Autodesk Inventor part; units mm, degrees
(part 2 of 2)
  arc A292 (23.8053, 31.1147) -> (23.1322, 30.5755) centre (29.291, 23.5772) ccw projected
  arc A293 (23.1322, 30.5755) -> (21.9307, 31.4483) centre (0, 0) ccw projected
  arc A294 (21.9307, 31.4483) -> (22.2356, 32.2552) centre (13.3718, 35.1431) ccw projected
  arc A295 (22.2356, 32.2552) -> (22.5669, 33.4681) centre (9.9788, 36.2544) ccw projected
  arc A296 (22.5669, 33.4681) -> (22.8546, 35.1883) centre (6.2739, 37.0778) ccw projected
  arc A297 (22.8546, 35.1883) -> (20.9772, 36.3388) centre (0, 0) ccw projected
  arc A298 (20.9772, 36.3388) -> (19.5752, 35.3014) centre (30.1882, 22.4231) ccw projected
  arc A299 (19.5752, 35.3014) -> (18.6448, 34.4556) centre (27.7726, 25.3503) ccw projected
  arc A300 (18.6448, 34.4556) -> (18.0643, 33.8177) centre (25.2421, 27.869) ccw projected
  arc A301 (18.0643, 33.8177) -> (16.7411, 34.4919) centre (0, 0) ccw projected
  arc A302 (16.7411, 34.4919) -> (16.916, 35.3365) centre (7.7096, 36.8023) ccw projected
  arc A303 (16.916, 35.3365) -> (17.0535, 36.5863) centre (4.1845, 37.3691) ccw projected
  arc A304 (17.0535, 36.5863) -> (17.0686, 38.3303) centre (0.3965, 37.6027) ccw projected
  arc A305 (17.0686, 38.3303) -> (15.0343, 39.1729) centre (0, 0) ccw projected
  arc A306 (15.0343, 39.1729) -> (13.8118, 37.9291) centre (26.3088, 26.8695) ccw projected
  arc A307 (13.8118, 37.9291) -> (13.0252, 36.9481) centre (23.4651, 29.3828) ccw projected
  arc A308 (13.0252, 36.9481) -> (12.5517, 36.2272) centre (20.5717, 31.4746) ccw projected
  arc A309 (12.5517, 36.2272) -> (11.1393, 36.6861) centre (0, 0) ccw projected
  arc A310 (11.1393, 36.6861) -> (11.1799, 37.5477) centre (1.8575, 37.5552) ccw projected
  arc A311 (11.1799, 37.5477) -> (11.1201, 38.8036) centre (-1.7129, 37.5636) ccw projected
  arc A312 (11.1201, 38.8036) -> (10.8623, 40.5285) centre (-5.4908, 37.2018) ccw projected
  arc A313 (10.8623, 40.5285) -> (8.7212, 41.0425) centre (0, 0) ccw projected
  arc A314 (8.7212, 41.0425) -> (7.7084, 39.6227) centre (21.7816, 30.6543) ccw projected
  arc A315 (7.7084, 39.6227) -> (7.0849, 38.5308) centre (18.5797, 32.6918) ccw projected
  arc A316 (7.0849, 38.5308) -> (6.73, 37.7447) centre (15.3947, 34.3052) ccw projected
  arc A317 (6.73, 37.7447) -> (5.2632, 37.977) centre (0, 0) ccw projected
  arc A318 (5.2632, 37.977) -> (5.1685, 38.8343) centre (-4.0403, 37.3834) ccw projected
  arc A319 (5.1685, 38.8343) -> (4.9158, 40.0547) centre (-7.568, 36.8332) ccw projected
  arc A320 (4.9158, 40.0547) -> (4.3885, 41.7288) centre (-11.2428, 35.8848) ccw projected
  arc A321 (4.3885, 41.7288) -> (2.1934, 41.9015) centre (0, 0) ccw projected
  arc A322 (2.1934, 41.9015) -> (1.4107, 40.3306) centre (16.718, 33.6843) ccw projected
  arc A323 (1.4107, 40.3306) -> (0.9701, 39.1647) centre (13.2368, 35.1958) ccw projected
  arc A324 (0.9701, 39.1647) -> (0.7425, 38.3328) centre (9.8386, 36.2911) ccw projected
  circle A325 centre (50, 0) radius 9
  line L1 (0, 0) -> (50, 0) construction
  circle A326 centre (50, 4.5) radius 2
  circle A327 centre (50, -4.5) radius 2
  line L2 (50, 4.5) -> (50, -4.5)
  line L3 (0, 0) -> (34.0976, 51.9877)
  line L4 (0, 0) -> (-5.7443, -48.4608)
  line L5 (21.9307, 31.4483) -> (2.9609, 2.5256)
  line L6 (-0.7425, -38.3328) -> (3.5093, -2.4629)
  line L7 (-0.7425, -38.3328) -> (7.758, -21.4754)
  line L8 (21.9307, 31.4483) -> (18.4149, 16.5287)
  line L9 (18.4149, 16.5287) -> (52.0246, 8.7693)
  line L10 (7.758, -21.4754) -> (52.4807, -8.6514)
  point P0 (37.977, 5.2632)
  point P1 (37.0268, -13.0827)
  point P2 (36.2778, 12.4048)
  point P3 (37.7447, 6.73)
  dimension "d2" = 6
  dimension "d3" = 6.13
  dimension "d5" = 7
  dimension "d37" = 18
  dimension "d38" = 50
  dimension "d39" = 4
  dimension "d40" = 4
  dimension "d42" = 9
  dimension "d43" = 56.74
  dimension "d44" = 153.5
  dimension "d45" = 20
  dimension "d46" = 20
  dimension "d47" = 13
  dimension "d48" = 16
  constraints: 22 end point, 6 centre point, 3 point on circle, 2 coincident, 2 parallel, 2 tangent, 2 vertical, 1 horizontal, 1 midpoint, 1 vertical alignment
  measures "d2" diameter of A0
  measures "d3" radial gap between concentric circles of A1 A2
  measures "d5" radial gap between concentric circles of A0 A3
  measures "d37" diameter of A325
  measures "d38" distance of L1.end L1.start
  measures "d39" diameter of A326
  measures "d40" diameter of A327
  measures "d42" distance of L2.start L2.end
  measures "d43" angle of L1 L3
  measures "d44" angle of L4 L3
  measures "d45" angle of L6 L7
  measures "d46" angle of L5 L8
  measures "d47" angle of L1 L9
  measures "d48" angle of L10 L1
extrude "押し出し6" cut sketch "Sketch2" against normal through all contours A0 L4 L3 | L3 L4 A0 | L8 A293 A292 A291 A290 A289 A288 A287 A286 A285 A284 A283 A282 A281 A280 A279 A278 A277 A276 A275 A274 A273 A272 A271 A270 A269 A268 A267 A266 A265 A264 A263 A262 A261 L9 A1 | A1 L9 L8 | L7 L10 A1 | A1 L10 A227 A226 A225 A224 A223 A222 A221 A220 A219 A218 A217 A216 A215 A214 A213 A212 A211 A210 A209 A208 A207 A206 A205 A204 A203 A202 A201 A200 A199 A198 A197 A196 A195 A194 A193 A192 A191 A190 A189 A188 A187 A186 A185 A184 A183 A182 A181 A180 A179 A178 A177 A176 A175 A174 A173 A172 A171 A170 A169 A168 A167 A166 A165 L7
extrude "押し出し7" add sketch "Sketch2" against normal blind 4 contours L9 A325 A249 A250 A251 A252 A4 A254 A255 A256 A257 A258 A259 A260 A261 | A227 A228 A229 A230 A231 A232 A233 A234 A235 A236 A237 A238 A239 A240 A241 A325 L10 | A325 A241 A242 A248 A249 | A325 A242 A243 A244 A245 A246 A247 A248
sketch "スケッチ6" plane through (0, 0, -4) normal (0, 0, -1) x (-1, 0, 0)
  circle A0 centre (-50, 4.5) radius 2 projected
  circle A1 centre (-50, -4.5) radius 2 projected
  line L0 (-7.758, -21.4754) -> (0.7425, -38.3328) projected
  arc A2 (0.7425, -38.3328) -> (0.9701, -39.1647) centre (9.8386, -36.2911) ccw projected
  arc A3 (0.9701, -39.1647) -> (1.4151, -40.3408) centre (13.2368, -35.1958) ccw projected
  arc A4 (1.4151, -40.3408) -> (2.1934, -41.9015) centre (16.718, -33.6843) ccw projected
  arc A5 (2.1934, -41.9015) -> (4.3885, -41.7288) centre (0, 0) ccw projected
  arc A6 (4.3885, -41.7288) -> (4.913, -40.0655) centre (-11.2428, -35.8848) ccw projected
  arc A7 (4.913, -40.0655) -> (5.1685, -38.8343) centre (-7.568, -36.8332) ccw projected
  arc A8 (5.1685, -38.8343) -> (5.2632, -37.977) centre (-4.0403, -37.3834) ccw projected
  arc A9 (5.2632, -37.977) -> (6.73, -37.7447) centre (0, 0) ccw projected
  arc A10 (6.73, -37.7447) -> (7.0849, -38.5308) centre (15.3947, -34.3052) ccw projected
  arc A11 (7.0849, -38.5308) -> (7.7084, -39.6227) centre (18.5797, -32.6918) ccw projected
  arc A12 (7.7084, -39.6227) -> (8.7212, -41.0425) centre (21.7816, -30.6543) ccw projected
  arc A13 (8.7212, -41.0425) -> (10.8623, -40.5285) centre (0, 0) ccw projected
  arc A14 (10.8623, -40.5285) -> (11.1201, -38.8036) centre (-5.4908, -37.2018) ccw projected
  arc A15 (11.1201, -38.8036) -> (11.1799, -37.5477) centre (-1.7129, -37.5636) ccw projected
  arc A16 (11.1799, -37.5477) -> (11.1393, -36.6861) centre (1.8575, -37.5552) ccw projected
  arc A17 (11.1393, -36.6861) -> (12.5517, -36.2272) centre (0, 0) ccw projected
  arc A18 (12.5517, -36.2272) -> (13.0252, -36.9481) centre (20.5717, -31.4746) ccw projected
  arc A19 (13.0252, -36.9481) -> (13.8118, -37.9291) centre (23.4651, -29.3828) ccw projected
  arc A20 (13.8118, -37.9291) -> (15.0343, -39.1729) centre (26.3088, -26.8695) ccw projected
  arc A21 (15.0343, -39.1729) -> (17.0686, -38.3303) centre (0, 0) ccw projected
  arc A22 (17.0686, -38.3303) -> (17.0535, -36.5863) centre (0.3965, -37.6027) ccw projected
  arc A23 (17.0535, -36.5863) -> (16.916, -35.3365) centre (4.1845, -37.3691) ccw projected
  arc A24 (16.916, -35.3365) -> (16.7411, -34.4919) centre (7.7096, -36.8023) ccw projected
  arc A25 (16.7411, -34.4919) -> (18.0643, -33.8177) centre (0, 0) ccw projected
  arc A26 (18.0643, -33.8177) -> (18.6448, -34.4556) centre (25.2421, -27.869) ccw projected
  arc A27 (18.6448, -34.4556) -> (19.5752, -35.3014) centre (27.7726, -25.3503) ccw projected
  arc A28 (19.5752, -35.3014) -> (20.9772, -36.3388) centre (30.1882, -22.4231) ccw projected
  arc A29 (20.9772, -36.3388) -> (22.8546, -35.1883) centre (0, 0) ccw projected
  arc A30 (22.8546, -35.1883) -> (22.5669, -33.4681) centre (6.2739, -37.0778) ccw projected
  arc A31 (22.5669, -33.4681) -> (22.2356, -32.2552) centre (9.9788, -36.2544) ccw projected
  arc A32 (22.2356, -32.2552) -> (21.9307, -31.4483) centre (13.3718, -35.1431) ccw projected
  arc A33 (21.9307, -31.4483) -> (23.1322, -30.5754) centre (0, 0) ccw projected
  arc A34 (23.1322, -30.5754) -> (23.8053, -31.1147) centre (29.291, -23.5771) ccw projected
  arc A35 (23.8053, -31.1147) -> (24.8565, -31.8046) centre (31.3964, -20.6936) ccw projected
  arc A36 (24.8565, -31.8046) -> (26.4036, -32.6098) centre (33.3243, -17.4245) ccw projected
  arc A37 (26.4036, -32.6098) -> (28.0779, -31.1798) centre (0, 0) ccw projected
  arc A38 (28.0779, -31.1798) -> (27.5246, -29.5259) centre (11.9969, -35.6398) ccw projected
  arc A39 (27.5246, -29.5259) -> (27.0076, -28.3796) centre (15.5273, -34.247) ccw projected
  arc A40 (27.0076, -28.3796) -> (26.5803, -27.6304) centre (18.7048, -32.6187) ccw projected
  arc A41 (26.5803, -27.6304) -> (27.6304, -26.5803) centre (0, 0) ccw projected
  arc A42 (27.6304, -26.5803) -> (28.3796, -27.0076) centre (32.6187, -18.7048) ccw projected
  arc A43 (28.3796, -27.0076) -> (29.5259, -27.5246) centre (34.247, -15.5273) ccw projected
  arc A44 (29.5259, -27.5246) -> (31.1798, -28.0779) centre (35.6398, -11.9969) ccw projected
  arc A45 (31.1798, -28.0779) -> (32.6098, -26.4036) centre (0, 0) ccw projected
  arc A46 (32.6098, -26.4036) -> (31.8046, -24.8565) centre (17.4245, -33.3243) ccw projected
  arc A47 (31.8046, -24.8565) -> (31.1147, -23.8053) centre (20.6936, -31.3964) ccw projected
  arc A48 (31.1147, -23.8053) -> (30.5754, -23.1322) centre (23.5771, -29.291) ccw projected
  arc A49 (30.5754, -23.1322) -> (31.4483, -21.9307) centre (0, 0) ccw projected
  arc A50 (31.4483, -21.9307) -> (32.2552, -22.2356) centre (35.1431, -13.3718) ccw projected
  arc A51 (32.2552, -22.2356) -> (33.4681, -22.5669) centre (36.2544, -9.9788) ccw projected
  arc A52 (33.4681, -22.5669) -> (35.1883, -22.8546) centre (37.0778, -6.2739) ccw projected
  arc A53 (35.1883, -22.8546) -> (36.3388, -20.9772) centre (0, 0) ccw projected
  arc A54 (36.3388, -20.9772) -> (35.3014, -19.5752) centre (22.4231, -30.1882) ccw projected
  arc A55 (35.3014, -19.5752) -> (34.4556, -18.6448) centre (25.3503, -27.7726) ccw projected
  arc A56 (34.4556, -18.6448) -> (33.8177, -18.0643) centre (27.869, -25.2421) ccw projected
  arc A57 (33.8177, -18.0643) -> (34.4919, -16.7411) centre (0, 0) ccw projected
  arc A58 (34.4919, -16.7411) -> (35.3365, -16.916) centre (36.8023, -7.7096) ccw projected
  arc A59 (35.3365, -16.916) -> (36.5863, -17.0535) centre (37.3691, -4.1845) ccw projected
  arc A60 (36.5863, -17.0535) -> (38.3303, -17.0686) centre (37.6027, -0.3965) ccw projected
  arc A61 (38.3303, -17.0686) -> (39.1729, -15.0343) centre (0, 0) ccw projected
  arc A62 (39.1729, -15.0343) -> (37.9291, -13.8118) centre (26.8695, -26.3088) ccw projected
  arc A63 (37.9291, -13.8118) -> (36.9481, -13.0252) centre (29.3828, -23.4651) ccw projected
  arc A64 (36.9481, -13.0252) -> (36.2272, -12.5517) centre (31.4746, -20.5717) ccw projected
  arc A65 (36.2272, -12.5517) -> (36.6861, -11.1393) centre (0, 0) ccw projected
  arc A66 (36.6861, -11.1393) -> (37.5477, -11.1799) centre (37.5552, -1.8575) ccw projected
  arc A67 (37.5477, -11.1799) -> (38.7926, -11.1212) centre (37.5636, 1.7129) ccw projected
  arc A68 (38.7926, -11.1212) -> (40.5285, -10.8623) centre (37.2018, 5.4908) ccw projected
  arc A69 (40.5285, -10.8623) -> (41.0425, -8.7212) centre (0, 0) ccw projected
  arc A70 (41.0425, -8.7212) -> (39.6227, -7.7084) centre (30.6543, -21.7816) ccw projected
  arc A71 (39.6227, -7.7084) -> (38.5308, -7.0849) centre (32.6918, -18.5797) ccw projected
  arc A72 (38.5308, -7.0849) -> (37.7447, -6.73) centre (34.3052, -15.3947) ccw projected
  arc A73 (37.7447, -6.73) -> (37.977, -5.2632) centre (0, 0) ccw projected
  arc A74 (37.977, -5.2632) -> (38.8343, -5.1685) centre (37.3834, 4.0403) ccw projected
  arc A75 (38.8343, -5.1685) -> (40.0655, -4.913) centre (36.8332, 7.568) ccw projected
  arc A76 (40.0655, -4.913) -> (41.7288, -4.3885) centre (35.8848, 11.2428) ccw projected
  arc A77 (41.7288, -4.3885) -> (41.9015, -2.1934) centre (0, 0) ccw projected
  arc A78 (41.9015, -2.1934) -> (40.3306, -1.4107) centre (33.6843, -16.718) ccw projected
  arc A79 (40.3306, -1.4107) -> (39.1647, -0.9701) centre (35.1958, -13.2368) ccw projected
  arc A80 (39.1647, -0.9701) -> (38.3328, -0.7425) centre (36.2911, -9.8386) ccw projected
  arc A81 (38.3328, -0.7425) -> (38.3328, 0.7425) centre (0, 0) ccw projected
  arc A82 (38.3328, 0.7425) -> (39.1647, 0.9701) centre (36.2911, 9.8386) ccw projected
  arc A83 (39.1647, 0.9701) -> (40.3306, 1.4107) centre (35.1958, 13.2368) ccw projected
  arc A84 (40.3306, 1.4107) -> (41.9015, 2.1934) centre (33.6843, 16.718) ccw projected
  arc A85 (41.9015, 2.1934) -> (41.7288, 4.3885) centre (0, 0) ccw projected
  arc A86 (41.7288, 4.3885) -> (40.0655, 4.913) centre (35.8848, -11.2428) ccw projected
  arc A87 (40.0655, 4.913) -> (38.8343, 5.1685) centre (36.8332, -7.568) ccw projected
  arc A88 (38.8343, 5.1685) -> (37.977, 5.2632) centre (37.3834, -4.0403) ccw projected
  arc A89 (37.977, 5.2632) -> (37.7447, 6.73) centre (0, 0) ccw projected
  arc A90 (37.7447, 6.73) -> (38.5308, 7.0849) centre (34.3052, 15.3947) ccw projected
  arc A91 (38.5308, 7.0849) -> (39.6227, 7.7084) centre (32.6918, 18.5797) ccw projected
  arc A92 (39.6227, 7.7084) -> (41.0425, 8.7212) centre (30.6543, 21.7816) ccw projected
  arc A93 (41.0425, 8.7212) -> (40.5285, 10.8623) centre (0, 0) ccw projected
  arc A94 (40.5285, 10.8623) -> (38.8036, 11.1201) centre (37.2018, -5.4908) ccw projected
  arc A95 (38.8036, 11.1201) -> (37.5477, 11.1799) centre (37.5636, -1.7129) ccw projected
  arc A96 (37.5477, 11.1799) -> (36.6861, 11.1393) centre (37.5552, 1.8575) ccw projected
  arc A97 (36.6861, 11.1393) -> (36.2272, 12.5517) centre (0, 0) ccw projected
  arc A98 (36.2272, 12.5517) -> (36.9365, 13.0169) centre (31.4746, 20.5717) ccw projected
  arc A99 (36.9365, 13.0169) -> (37.9291, 13.8118) centre (29.3828, 23.4651) ccw projected
  arc A100 (37.9291, 13.8118) -> (39.1729, 15.0343) centre (26.8695, 26.3088) ccw projected
  arc A101 (39.1729, 15.0343) -> (38.3303, 17.0686) centre (0, 0) ccw projected
  arc A102 (38.3303, 17.0686) -> (36.5863, 17.0535) centre (37.6027, 0.3965) ccw projected
  arc A103 (36.5863, 17.0535) -> (35.3365, 16.916) centre (37.3691, 4.1845) ccw projected
  arc A104 (35.3365, 16.916) -> (34.4919, 16.7411) centre (36.8023, 7.7096) ccw projected
  arc A105 (34.4919, 16.7411) -> (33.8177, 18.0643) centre (0, 0) ccw projected
  arc A106 (33.8177, 18.0643) -> (34.4556, 18.6448) centre (27.869, 25.2421) ccw projected
  arc A107 (34.4556, 18.6448) -> (35.3014, 19.5752) centre (25.3503, 27.7726) ccw projected
  arc A108 (35.3014, 19.5752) -> (36.3388, 20.9772) centre (22.4231, 30.1882) ccw projected
  arc A109 (36.3388, 20.9772) -> (35.1883, 22.8546) centre (0, 0) ccw projected
  arc A110 (35.1883, 22.8546) -> (33.4681, 22.5669) centre (37.0778, 6.2739) ccw projected
  arc A111 (33.4681, 22.5669) -> (32.2552, 22.2356) centre (36.2544, 9.9788) ccw projected
  arc A112 (32.2552, 22.2356) -> (31.4483, 21.9307) centre (35.1431, 13.3718) ccw projected
  arc A113 (31.4483, 21.9307) -> (30.5755, 23.1322) centre (0, 0) ccw projected
  arc A114 (30.5755, 23.1322) -> (31.1147, 23.8053) centre (23.5772, 29.291) ccw projected
  arc A115 (31.1147, 23.8053) -> (31.8046, 24.8565) centre (20.6936, 31.3964) ccw projected
  arc A116 (31.8046, 24.8565) -> (32.6098, 26.4036) centre (17.4245, 33.3243) ccw projected
  arc A117 (32.6098, 26.4036) -> (31.1798, 28.0779) centre (0, 0) ccw projected
  arc A118 (31.1798, 28.0779) -> (29.5259, 27.5246) centre (35.6398, 11.9969) ccw projected
  arc A119 (29.5259, 27.5246) -> (28.3796, 27.0076) centre (34.247, 15.5273) ccw projected
  arc A120 (28.3796, 27.0076) -> (27.6304, 26.5803) centre (32.6187, 18.7048) ccw projected
  arc A121 (27.6304, 26.5803) -> (26.5803, 27.6304) centre (0, 0) ccw projected
  arc A122 (26.5803, 27.6304) -> (27.0076, 28.3796) centre (18.7048, 32.6187) ccw projected
  arc A123 (27.0076, 28.3796) -> (27.5246, 29.5259) centre (15.5273, 34.247) ccw projected
  arc A124 (27.5246, 29.5259) -> (28.0779, 31.1798) centre (11.9969, 35.6398) ccw projected
  arc A125 (28.0779, 31.1798) -> (26.4036, 32.6098) centre (0, 0) ccw projected
  arc A126 (26.4036, 32.6098) -> (24.8565, 31.8046) centre (33.3243, 17.4245) ccw projected
  arc A127 (24.8565, 31.8046) -> (23.8053, 31.1147) centre (31.3964, 20.6936) ccw projected
  arc A128 (23.8053, 31.1147) -> (23.1322, 30.5755) centre (29.291, 23.5772) ccw projected
  arc A129 (23.1322, 30.5755) -> (21.9307, 31.4483) centre (0, 0) ccw projected
  arc A130 (21.9307, 31.4483) -> (22.2356, 32.2552) centre (13.3718, 35.1431) ccw projected
  arc A131 (22.2356, 32.2552) -> (22.5669, 33.4681) centre (9.9788, 36.2544) ccw projected
  arc A132 (22.5669, 33.4681) -> (22.8546, 35.1883) centre (6.2739, 37.0778) ccw projected
  arc A133 (22.8546, 35.1883) -> (20.9772, 36.3388) centre (0, 0) ccw projected
  arc A134 (20.9772, 36.3388) -> (19.5752, 35.3014) centre (30.1882, 22.4231) ccw projected
  arc A135 (19.5752, 35.3014) -> (18.6448, 34.4556) centre (27.7726, 25.3503) ccw projected
  arc A136 (18.6448, 34.4556) -> (18.0643, 33.8177) centre (25.2421, 27.869) ccw projected
  arc A137 (18.0643, 33.8177) -> (16.7411, 34.4919) centre (0, 0) ccw projected
  arc A138 (16.7411, 34.4919) -> (16.916, 35.3365) centre (7.7096, 36.8023) ccw projected
  arc A139 (16.916, 35.3365) -> (17.0535, 36.5863) centre (4.1845, 37.3691) ccw projected
  arc A140 (17.0535, 36.5863) -> (17.0686, 38.3303) centre (0.3965, 37.6027) ccw projected
  arc A141 (17.0686, 38.3303) -> (15.0343, 39.1729) centre (0, 0) ccw projected
  arc A142 (15.0343, 39.1729) -> (13.8118, 37.9291) centre (26.3088, 26.8695) ccw projected
  arc A143 (13.8118, 37.9291) -> (13.0252, 36.9481) centre (23.4651, 29.3828) ccw projected
  arc A144 (13.0252, 36.9481) -> (12.5517, 36.2272) centre (20.5717, 31.4746) ccw projected
  arc A145 (12.5517, 36.2272) -> (11.1393, 36.6861) centre (0, 0) ccw projected
  arc A146 (11.1393, 36.6861) -> (11.1799, 37.5477) centre (1.8575, 37.5552) ccw projected
  arc A147 (11.1799, 37.5477) -> (11.1212, 38.7926) centre (-1.7129, 37.5636) ccw projected
  arc A148 (11.1212, 38.7926) -> (10.8623, 40.5285) centre (-5.4908, 37.2018) ccw projected
  arc A149 (10.8623, 40.5285) -> (8.7212, 41.0425) centre (0, 0) ccw projected
  arc A150 (8.7212, 41.0425) -> (7.7084, 39.6227) centre (21.7816, 30.6543) ccw projected
  arc A151 (7.7084, 39.6227) -> (7.0849, 38.5308) centre (18.5797, 32.6918) ccw projected
  arc A152 (7.0849, 38.5308) -> (6.73, 37.7447) centre (15.3947, 34.3052) ccw projected
  arc A153 (6.73, 37.7447) -> (5.2632, 37.977) centre (0, 0) ccw projected
  arc A154 (5.2632, 37.977) -> (5.1685, 38.8343) centre (-4.0403, 37.3834) ccw projected
  arc A155 (5.1685, 38.8343) -> (4.913, 40.0655) centre (-7.568, 36.8332) ccw projected
  arc A156 (4.913, 40.0655) -> (4.3885, 41.7288) centre (-11.2428, 35.8848) ccw projected
  arc A157 (4.3885, 41.7288) -> (2.1934, 41.9015) centre (0, 0) ccw projected
  arc A158 (2.1934, 41.9015) -> (1.4151, 40.3408) centre (16.718, 33.6843) ccw projected
  arc A159 (1.4151, 40.3408) -> (0.9657, 39.1511) centre (13.2368, 35.1958) ccw projected
  arc A160 (0.9657, 39.1511) -> (0.7425, 38.3328) centre (9.8386, 36.2911) ccw projected
  arc A161 (0.7425, 38.3328) -> (-0.7425, 38.3328) centre (0, 0) ccw projected
  arc A162 (-0.7425, 38.3328) -> (-0.9701, 39.1647) centre (-9.8386, 36.2911) ccw projected
  arc A163 (-0.9701, 39.1647) -> (-1.4107, 40.3306) centre (-13.2368, 35.1958) ccw projected
  arc A164 (-1.4107, 40.3306) -> (-2.1934, 41.9015) centre (-16.718, 33.6843) ccw projected
  arc A165 (-2.1934, 41.9015) -> (-4.3885, 41.7288) centre (0, 0) ccw projected
  arc A166 (-4.3885, 41.7288) -> (-4.9158, 40.0547) centre (11.2428, 35.8848) ccw projected
  arc A167 (-4.9158, 40.0547) -> (-5.1685, 38.8343) centre (7.568, 36.8332) ccw projected
  arc A168 (-5.1685, 38.8343) -> (-5.2632, 37.977) centre (4.0403, 37.3834) ccw projected
  arc A169 (-5.2632, 37.977) -> (-6.73, 37.7447) centre (0, 0) ccw projected
  arc A170 (-6.73, 37.7447) -> (-7.0849, 38.5308) centre (-15.3947, 34.3052) ccw projected
  arc A171 (-7.0849, 38.5308) -> (-7.7084, 39.6227) centre (-18.5797, 32.6918) ccw projected
  arc A172 (-7.7084, 39.6227) -> (-8.7212, 41.0425) centre (-21.7816, 30.6543) ccw projected
  arc A173 (-8.7212, 41.0425) -> (-10.8623, 40.5285) centre (0, 0) ccw projected
  arc A174 (-10.8623, 40.5285) -> (-11.1201, 38.8036) centre (5.4908, 37.2018) ccw projected
  arc A175 (-11.1201, 38.8036) -> (-11.1799, 37.5477) centre (1.7129, 37.5636) ccw projected
  arc A176 (-11.1799, 37.5477) -> (-11.1393, 36.6861) centre (-1.8575, 37.5552) ccw projected
  arc A177 (-11.1393, 36.6861) -> (-12.5517, 36.2272) centre (0, 0) ccw projected
  arc A178 (-12.5517, 36.2272) -> (-13.0252, 36.9481) centre (-20.5717, 31.4746) ccw projected
  arc A179 (-13.0252, 36.9481) -> (-13.8118, 37.9291) centre (-23.4651, 29.3828) ccw projected
  arc A180 (-13.8118, 37.9291) -> (-15.0343, 39.1729) centre (-26.3088, 26.8695) ccw projected
  arc A181 (-15.0343, 39.1729) -> (-17.0686, 38.3303) centre (0, 0) ccw projected
  arc A182 (-17.0686, 38.3303) -> (-17.0535, 36.5863) centre (-0.3965, 37.6027) ccw projected
  arc A183 (-17.0535, 36.5863) -> (-16.916, 35.3365) centre (-4.1845, 37.3691) ccw projected
  arc A184 (-16.916, 35.3365) -> (-16.7411, 34.4919) centre (-7.7096, 36.8023) ccw projected
  arc A185 (-16.7411, 34.4919) -> (-18.0643, 33.8177) centre (0, 0) ccw projected
  arc A186 (-18.0643, 33.8177) -> (-18.6448, 34.4556) centre (-25.2421, 27.869) ccw projected
  arc A187 (-18.6448, 34.4556) -> (-19.5752, 35.3014) centre (-27.7726, 25.3503) ccw projected
  arc A188 (-19.5752, 35.3014) -> (-20.9772, 36.3388) centre (-30.1882, 22.4231) ccw projected
  arc A189 (-20.9772, 36.3388) -> (-22.8546, 35.1883) centre (0, 0) ccw projected
  arc A190 (-22.8546, 35.1883) -> (-22.5669, 33.4681) centre (-6.2739, 37.0778) ccw projected
  arc A191 (-22.5669, 33.4681) -> (-22.2356, 32.2552) centre (-9.9788, 36.2544) ccw projected
  arc A192 (-22.2356, 32.2552) -> (-21.9307, 31.4483) centre (-13.3718, 35.1431) ccw projected
  line L1 (-21.9307, 31.4483) -> (-18.4149, 16.5287) projected
  line L2 (-18.4149, 16.5287) -> (-52.0246, 8.7693) projected
  arc A193 (-52.0246, 8.7693) -> (-52.4807, -8.6514) centre (-50, 0) ccw projected
  line L3 (-52.4807, -8.6514) -> (-7.758, -21.4754) projected
  circle A194 centre (0, 0) radius 3 projected
  circle A195 centre (0, 0) radius 37.6026
  circle A196 centre (0, 0) radius 32.6026
  line L4 (-16.9189, 27.869) -> (-7.0849, 10.0792)
  circle A197 centre (0, 0) radius 12.3201
  dimension "d53" = 5
  constraints: 2 coincident, 2 end point, 9 other
body "Solid1"
